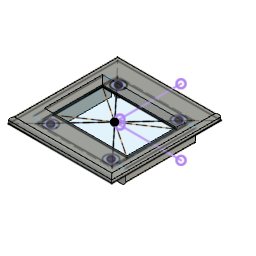
PMS5003-enclosure v2 (Autodesk Fusion 360 archive; units mm, degrees)
design "OLED display bezel"
Autodesk Fusion 360 part; units mm, degrees
sketch "Sketch1" plane through (0, 0, 0) normal (0, 0, 1) x (1, 0, 0)
  line L0 (12.5, -13.5) -> (-12.5, -13.5)
  line L1 (-12.5, -13.5) -> (-12.5, 13.5)
  line L2 (-12.5, 13.5) -> (12.5, 13.5)
  line L3 (12.5, 13.5) -> (12.5, -13.5)
  line L4 (12.5, -13.5) -> (-12.5, 13.5) construction
  line L5 (-12.5, -13.5) -> (12.5, 13.5) construction
  circle A0 centre (10.2493, 11.5) radius 1.35
  line L6 (1.75, 0) -> (22.5, 0)
  circle A1 centre (10.2493, -11.5) radius 1.35
  line L7 (0, 1.75) -> (0, 22.5)
  circle A2 centre (-10.2507, 11.5) radius 1.3608
  circle A3 centre (-10.2507, -11.5) radius 1.3608
  line L8 (12.5, -8.35) -> (-12.5, -8.35)
  line L9 (-12.5, -8.35) -> (-12.5, 8.35)
  line L10 (-12.5, 8.35) -> (12.5, 8.35)
  line L11 (12.5, 8.35) -> (12.5, -8.35)
  line L12 (12.5, -8.35) -> (-12.5, 8.35) construction
  line L13 (-12.5, -8.35) -> (12.5, 8.35) construction
  dimension "d1" = 25
  dimension "d2" = 27
  dimension "d5" = 2.7
  dimension "d6" = 16.7
  dimension "d37" = 20.5
  dimension "d38" = 23
  dimension "d39" = 23
  constraint horizontal L0
  constraint perpendicular L0 L1
  constraint parallel L0 L2
  constraint parallel L1 L3
  constraint coincident L4 origin
  constraint coincident L5 origin
  constraint horizontal L8
  constraint perpendicular L8 L9
  constraint parallel L8 L10
  constraint parallel L9 L11
  constraint coincident L12 origin
  constraint coincident L13 origin
  constraint symmetric L6 A2 A3
  constraint symmetric A0 L6 A1
  measures "d1" distance of L1.end L2.end
  measures "d2" distance of L0.end L1.end
  measures "d5" diameter of A0
  measures "d6" distance of L8.end L9.end
  measures "d37" distance of A0.centre A2.centre
  measures "d38" distance of A0.centre A1.centre
  measures "d39" distance of A2.centre A3.centre
extrude "Extrude1" add sketch "Sketch1" against normal blind 1.2 makes body 1
extrude "Extrude2" add sketch "Sketch1" along normal blind 2.05 contours L1 L3 L8 L9 L10 L11 bodies 1
sketch "Sketch2" plane through (0, 0, 0) normal (0, 0, 1) x (1, 0, 0)
  line L0 (17.5, -18.5) -> (-17.5, -18.5)
  line L1 (-17.5, -18.5) -> (-17.5, 18.5)
  line L2 (-17.5, 18.5) -> (17.5, 18.5)
  line L3 (17.5, 18.5) -> (17.5, -18.5)
  line L4 (17.5, -18.5) -> (-17.5, 18.5) construction
  line L5 (-17.5, -18.5) -> (17.5, 18.5) construction
  line L6 (-12.5, 8.35) -> (12.5, 8.35)
  line L7 (12.5, 8.35) -> (12.5, -8.35)
  line L8 (12.5, -8.35) -> (-12.5, -8.35)
  line L9 (-12.5, -8.35) -> (-12.5, 8.35)
  line L10 (-12.5, 8.35) -> (12.5, -8.35) construction
  line L11 (12.5, 8.35) -> (-12.5, -8.35) construction
  line L12 (13, 14) -> (-13, 14) construction
  line L13 (-13, 14) -> (-13, -14) construction
  line L14 (-13, -14) -> (13, -14) construction
  line L15 (13, -14) -> (13, 14) construction
  line L16 (13, 14) -> (-13, -14) construction
  line L17 (-13, 14) -> (13, -14) construction
  line L18 (-13, -11.9651) -> (-13, 11.9437)
  line L19 (-13, 11.9437) -> (-15.5, 11.9437)
  line L20 (-15.5, 11.9437) -> (-15.5, -11.9651)
  line L21 (-15.5, -11.9651) -> (-13, -11.9651)
  line L22 (0, 1.75) -> (0, 22.5)
  line L23 (13, -11.9651) -> (13, 11.9437)
  line L24 (15.5, 11.9437) -> (15.5, -11.9651)
  line L25 (15.5, -11.9651) -> (13, -11.9651)
  line L26 (13, 11.9437) -> (15.5, 11.9437)
  circle A0 centre (10.2493, -11.5) radius 1.35 construction
  circle A1 centre (-10.2507, -11.5) radius 1.3608 construction
  circle A2 centre (-10.2507, 11.5) radius 1.3608 construction
  circle A3 centre (10.2493, 11.5) radius 1.35 construction
  circle A4 centre (-10.2507, -11.5) radius 1
  line L27 (1.75, 0) -> (22.5, 0)
  circle A5 centre (-10.2507, 11.5) radius 1
  circle A6 centre (10.2507, 11.5) radius 1
  circle A7 centre (10.2507, -11.5) radius 1
  circle A8 centre (-10.2507, -11.5) radius 2.0492
  circle A9 centre (-10.2507, 11.5) radius 2.0492
  circle A10 centre (-10.2507, 11.5) radius 2.0492
  circle A11 centre (10.2507, 11.5) radius 2.0492
  circle A12 centre (10.2507, -11.5) radius 2.0492
  dimension "d15" = 35
  dimension "d16" = 37
  dimension "d17" = 25
  dimension "d18" = 16.7
  dimension "d24" = 26
  dimension "d25" = 28
  dimension "d26" = 2.5
  dimension "d31" = 2
  constraint horizontal L0
  constraint perpendicular L0 L1
  constraint parallel L0 L2
  constraint parallel L1 L3
  constraint coincident L4 origin
  constraint coincident L5 origin
  constraint horizontal L6
  constraint perpendicular L6 L7
  constraint parallel L6 L8
  constraint parallel L7 L9
  constraint coincident L10 origin
  constraint coincident L11 origin
  constraint horizontal L12
  constraint perpendicular L12 L13
  constraint parallel L12 L14
  constraint parallel L13 L15
  constraint coincident L16 origin
  constraint coincident L17 origin
  constraint perpendicular L18 L19
  constraint parallel L18 L20
  constraint parallel L19 L21
  constraint coincident L13 L18.end
  constraint parallel L13 L18
  constraint symmetric L18.start L22 L23.start
  constraint symmetric L18.end L22 L23.end
  constraint symmetric L19.end L22 L24.start
  constraint symmetric L20.end L22 L24.end
  constraint concentric A1 A4
  constraint symmetric A4 L27 A5
  constraint symmetric L22 A4 A7
  constraint symmetric L22 A5 A6
  constraint concentric A4 A8
  constraint symmetric L27 A8 A9
  constraint symmetric L27 A8 A10
  constraint symmetric L22 A8 A12
  constraint symmetric L22 A9 A11
  measures "d15" distance of L1.end L2.end
  measures "d16" distance of L0.end L1.end
  measures "d17" distance of L7.end L8.end
  measures "d18" distance of L6.end L7.end
  measures "d24" distance of L13.end L14.end
  measures "d25" distance of L12.end L13.end
  measures "d26" distance of L18.start L20.end
  measures "d31" diameter of A4
extrude "Extrude3" add sketch "Sketch2" along normal blind 2 separate body contours L0 L1 L2 L3 L6 L7 L8 L9 L22 L23 L24 L25 L27 | L2 L3 L6 L7 L22 L23 L24 L26 L27 | L23 L24 L26 L27 | L23 L24 L25 L27 | L18 L19 L20 L21 | A4 | A5 | A6 | A7 | A8 | A9 A10 | A11 | A12 makes body 2
move_body "Move1" bodies 1 to x (1, 0, 0) y (0, 1, 0) z (0, 0, 1) at (0, 0, -2)
chamfer "Chamfer1" distance 1.5 angle 45 4 edges at (0, 8.35, 2) (-12.5, 0, 2) (0, -8.35, 2) (12.5, 0, 2) on bodies 2
extrude "Extrude4" add sketch "Sketch2" against normal blind 5 contours L23 L24 L26 L27 | L23 L24 L25 L27 | L18 L19 L20 L21 bodies 2
fillet "Fillet1" radius 1 2 edges at (15.5, -0.0107, -5) (-15.5, -0.0107, -5) on bodies 2
fillet "Fillet2" radius 1 4 edges at (0, 18.5, 2) (-17.5, 0, 2) (0, -18.5, 2) (17.5, 0, 2) on bodies 2
extrude "Extrude6" add sketch "Sketch2" against normal blind 3.5 contours A4 | A5 | A6 | A7 bodies 2
fillet "Fillet3" radius 0.5 4 edges at (-11.183, -11.1384, -3.5) (9.3183, -11.1384, -3.5) (9.3183, 11.8616, -3.5) (-11.183, 11.8616, -3.5) on bodies 2
hidden bodies 1
equation "d1 = pcb_width"
equation "d2 = pcb_height"
equation "d5 = drill_diameter"
equation "pcb_width = 25 mm"
equation "pcb_height = 27 mm"
equation "oled_width = 16.7 mm"
equation "drill_diameter = 2.70 mm"
equation "d15 = pcb_width + 10 mm"
equation "d16 = pcb_height + 10 mm"
equation "d17 = pcb_width"
equation "d18 = oled_width"
equation "d24 = pcb_width + 1 mm"
equation "d25 = pcb_height + 1 mm"
named bodies: "oled-screen", "bezel"
